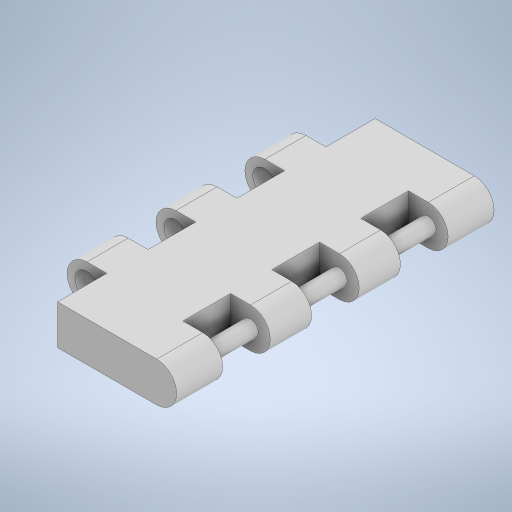
# Autodesk Inventor part: chain_link
Saved by Autodesk Inventor 2023 (Build 270158000, 158)
## iProperties
Created: 2023-05-24
Part Number: chain_link
Material: Generic
Document SubType Name: Modeling
Designer: nemes
Density: 1 g/cm^3
Appearance: Default
Author: nemes
Autodesk Inventor part; units mm, degrees
ref_plane "YZ Plane" through (0, 0, 0) normal (1, 0, 0) x (0, 1, 0)
ref_plane "XZ Plane" through (0, 0, 0) normal (0, 1, 0) x (-1, 0, 0)
ref_plane "XY Plane" through (0, 0, 0) normal (0, 0, 1) x (1, 0, 0)
sketch "Sketch1" plane through (0, 0, 0) normal (0, 0, 1) x (1, 0, 0)
  arc A0 (-3.75, -2.5) -> (-3.75, -5) centre (-3.75, -3.75) ccw
  arc A1 (3.75, -5) -> (3.75, -2.5) centre (3.75, -3.75) ccw
  line L0 (-3.75, -2.5) -> (3.75, -2.5)
  line L1 (3.75, -5) -> (-3.75, -5)
  circle A2 centre (-3.75, -3.75) radius 0.75
  circle A3 centre (3.75, -3.75) radius 0.5
  circle A4 centre (3.75, -3.75) radius 0.5
  point P0 (0, 0)
  dimension "d0" = 2.5
  dimension "d1" = 5
  dimension "d4" = 7.5
  dimension "d5" = 3.75
  dimension "d6" = 1.5
  dimension "d7" = 1
  dimension "d77" = 1
  constraints: 5 centre point, 4 end point, 4 point on circle, 4 tangent, 3 coincident, 2 concentric, 1 horizontal, 1 parallel
  measures "d0" distance between parallel lines of L1 L0
  measures "d1" distance from line of L1 point (0, 0)
  measures "d4" distance of point (3.75, -3.75) point (-3.75, -3.75)
  measures "d5" horizontal distance of point (0, 0) A0.centre
  measures "d6" diameter of A2
  measures "d7" diameter of A3
  measures "d77" diameter of A4
extrude "Extrusion1" add sketch "Sketch1" along normal blind 20
sketch "Sketch3" plane through (0, 0, 0) normal (0, 1, 0) x (-1, 0, 0)
  line L0 (5, 0) -> (3.75, 0) projected
  line L1 (-3.75, 0) -> (3.75, 0) projected
  line L2 (5, 16.9) -> (2.5, 16.9)
  line L3 (2.5, 16.9) -> (2.5, 20)
  line L4 (2.5, 20) -> (5, 20)
  line L5 (5, 20) -> (5, 16.9)
  line L6 (5, 14.3) -> (2.5, 14.3)
  line L7 (2.5, 14.3) -> (2.5, 11.3)
  line L8 (2.5, 11.3) -> (5, 11.3)
  line L9 (5, 11.3) -> (5, 14.3)
  line L10 (5, 5.7) -> (2.5, 5.7)
  line L11 (2.5, 5.7) -> (2.5, 8.7)
  line L12 (2.5, 8.7) -> (5, 8.7)
  line L13 (5, 8.7) -> (5, 5.7)
  line L14 (5, 0) -> (2.5, 0)
  line L15 (2.5, 0) -> (2.5, 3.1)
  line L16 (2.5, 3.1) -> (5, 3.1)
  line L17 (5, 3.1) -> (5, 0)
  line L18 (-2.5, 2.9) -> (-5, 2.9)
  line L19 (-5, 2.9) -> (-5, 5.9)
  line L20 (-5, 5.9) -> (-2.5, 5.9)
  line L21 (-2.5, 5.9) -> (-2.5, 2.9)
  line L22 (-2.5, 8.5) -> (-5, 8.5)
  line L23 (-5, 8.5) -> (-5, 11.5)
  line L24 (-5, 11.5) -> (-2.5, 11.5)
  line L25 (-2.5, 11.5) -> (-2.5, 8.5)
  line L26 (-2.5, 14.1) -> (-5, 14.1)
  line L27 (-5, 14.1) -> (-5, 17.1)
  line L28 (-5, 17.1) -> (-2.5, 17.1)
  line L29 (-2.5, 17.1) -> (-2.5, 14.1)
  point P0 (0, 0)
  point P1 (0, 0)
  point P2 (0, 0)
  point P3 (0, 0)
  point P4 (0, 0)
  point P5 (0, 0)
  point P6 (0, 0)
  point P7 (0, 0)
  point P8 (0, 0)
  dimension "d49" = 2.5
  dimension "d50" = 2.5
  dimension "d52" = 3.1
  dimension "d53" = 3.1
  dimension "d54" = 3
  dimension "d55" = 3
  dimension "d56" = 3
  dimension "d57" = 3
  dimension "d58" = 3
  dimension "d72" = 10
  dimension "d73" = 5
  dimension "d74" = 0
  dimension "d80" = 0.2
  dimension "d81" = 0.2
  dimension "d82" = 0.2
  dimension "d83" = 0.2
  dimension "d84" = 0.2
  dimension "d85" = 0.2
  constraints: 56 end point, 14 parallel, 10 point on line, 7 horizontal, 7 perpendicular, 7 other
  measures "d49" distance of L14.start L14.end
  measures "d50" distance of L18.start L18.end
  measures "d52" distance of L16.end L14.start
  measures "d53" distance of L4.end L2.start
  measures "d54" distance of L26.end L27.end
  measures "d55" distance of L8.end L6.start
  measures "d56" distance of L22.end L23.end
  measures "d57" distance of L12.end L10.start
  measures "d58" distance of L18.end L19.end
  measures "d72" distance between parallel lines of L19 L17
  measures "d73" distance from line of L5 point (0, 0)
  measures "d74" distance from line of point (0, 0) L14
  measures "d80" distance between parallel lines of L16 L18
  measures "d81" distance between parallel lines of L20 L10
  measures "d82" distance between parallel lines of L12 L22
  measures "d83" distance between parallel lines of L24 L8
  measures "d84" distance between parallel lines of L26 L6
  measures "d85" distance between parallel lines of L28 L2
extrude "Extrusion2" cut sketch "Sketch3" against normal blind 20
extrude "Extrusion3" add sketch "Sketch1" along normal blind 20 contours A3
body "Solid1"
